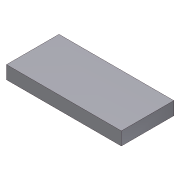
# Autodesk Inventor part: Tantalum_4x9x1
Saved by Autodesk Inventor 2014 SP1 (Build 180222100, 222)
## iProperties
Created: 2014-03-24
Part Number: Tantalum_4x9x1
Material: Tantalum
Document SubType Name: Modeling
Designer: Robert Davis
Mass: 0.58415 g
Surface Area: 0.955 cm^2
Volume: 0.035 cm^3
Density: 16.69 g/cm^3
Appearance: Steel
Author: Robert Davis
Autodesk Inventor part; units mm, degrees
ref_plane "YZ Plane" through (0, 0, 0) normal (1, 0, 0) x (0, 1, 0)
ref_plane "XZ Plane" through (0, 0, 0) normal (0, 1, 0) x (-1, 0, 0)
ref_plane "XY Plane" through (0, 0, 0) normal (0, 0, 1) x (1, 0, 0)
sketch "Sketch1" plane through (0, 0, 0) normal (0, 0, 1) x (1, 0, 0)
  line L0 (0, 1.5119) -> (0, 0)
  line L1 (0, 0) -> (2.1802, 0)
  line L2 (4.375, 2) -> (4.375, -2)
  line L3 (4.375, -2) -> (-4.375, -2)
  line L4 (-4.375, -2) -> (-4.375, 2)
  line L5 (-4.375, 2) -> (4.375, 2)
  dimension "d0" = 4
  dimension "d1" = 8.75
  constraints: 12 end point, 3 vertical, 2 horizontal, 1 coincident, 2 other
  measures "d0" distance of L3.end L4.end
  measures "d1" distance of L4.end L2.start
extrude "Extrusion1" add sketch "Sketch1" along normal mid plane 1
body "Solid1"
